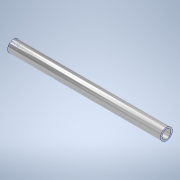
# Autodesk Inventor part: 上下直動_ベアリングシャフト
Saved by Autodesk Inventor 2020.3 (Build 243373000, 373)
## iProperties
Created: 2020-07-05
Part Number: 上下直動_ベアリングシャフト
Material: アルミニウム 6061
Document SubType Name: Modeling
Designer: totot
Mass: 0.497275 g
Surface Area: 7.47699 cm^2
Volume: 0.184176 cm^3
Density: 2.7 g/cm^3
Appearance: アルミニウム - フラット
Author: totot
Autodesk Inventor part; units mm, degrees
ref_plane "YZ Plane" through (0, 0, 0) normal (1, 0, 0) x (0, 1, 0)
ref_plane "XZ Plane" through (0, 0, 0) normal (0, 1, 0) x (-1, 0, 0)
ref_plane "XY Plane" through (0, 0, 0) normal (0, 0, 1) x (1, 0, 0)
sketch "スケッチ1" plane through (0, 0, 0) normal (1, 0, 0) x (0, 1, 0)
  circle A0 centre (0, 0) radius 2
  circle A1 centre (0, 0) radius 1.5
  dimension "d0" = 4
  dimension "d1" = 3
  constraints: 2 centre point, 2 coincident
  measures "d0" diameter of A0
  measures "d1" diameter of A1
extrude "押し出し1" add sketch "スケッチ1" along normal blind 51.5
